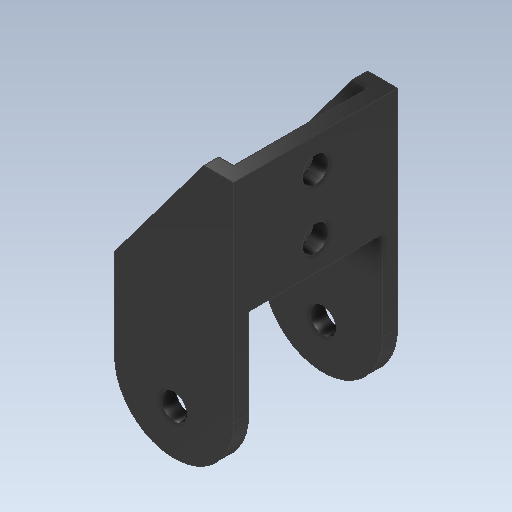
# Autodesk Inventor part: Kit de Sujeción 2
Saved by Autodesk Inventor 2020 (Build 240168000, 168)
## iProperties
Created: 2020-07-05
Part Number: Kit de Sujeción 2
Material: Genérico
Document SubType Name: Modeling
Designer: Pipi
Density: 1 g/cm^3
Appearance: Brillante - Negro
Author: Pipi
Autodesk Inventor part; units mm, degrees
ref_plane "YZ Plane" through (0, 0, 0) normal (1, 0, 0) x (0, 1, 0)
ref_plane "XZ Plane" through (0, 0, 0) normal (0, 1, 0) x (-1, 0, 0)
ref_plane "XY Plane" through (0, 0, 0) normal (0, 0, 1) x (1, 0, 0)
sketch "Boceto1" plane through (0, 0, 0) normal (0, 1, 0) x (-1, 0, 0)
  line L0 (10.3005, 0.2018) -> (-1.6995, 0.2018)
  line L1 (-1.6995, 0.2018) -> (-1.6995, 18.2018)
  line L2 (-1.6995, 18.2018) -> (10.3005, 18.2018)
  line L3 (12.3005, 20.2018) -> (-3.6995, 20.2018)
  line L4 (-3.6995, 20.2018) -> (-3.6995, -1.7982)
  line L5 (-3.6995, -1.7982) -> (12.3005, -1.7982)
  line L6 (10.3005, 18.2018) -> (12.3005, 18.2018)
  line L7 (10.3005, 0.2018) -> (12.3005, 0.2018)
  line L8 (12.3005, -1.7982) -> (12.3005, 0.2018)
  line L9 (12.3005, 18.2018) -> (12.3005, 20.2018)
  point P0 (0, 0)
  point P1 (0, 0)
  dimension "d0" = 18
  dimension "d1" = 12
  constraints: 20 end point, 10 perpendicular, 2 other
  measures "d0" distance of L2.end L0.start
  measures "d1" distance of L0.start L0.end
extrude "Extrusión1" add sketch "Boceto1" along normal blind 28
sketch "Boceto4" plane through (1.6995, 0, 0.2018) normal (-1, 0, 0) x (0, 0, 1)
  line L0 (18, 0) -> (18, 28) projected
  line L1 (18, 28) -> (18, 12)
  line L2 (18, 12) -> (0, 12)
  line L3 (0, 0) -> (0, 28) projected
  line L4 (18, 28) -> (0, 28)
  line L5 (0, 28) -> (0, 12)
  line L6 (20, 28) -> (-2, 28) projected
  line L7 (9, 28) -> (9, 12)
  circle A0 centre (9, 24) radius 1.75
  circle A1 centre (9, 16) radius 1.75
  line L8 (18, 12) -> (18, 0)
  line L9 (0, 0) -> (18, 0) projected
  line L10 (0, 0) -> (0, 12)
  line L11 (18, 0) -> (0, 0)
  point P0 (-0.2018, 0)
  dimension "d14" = 16
  dimension "d15" = 3.5
  dimension "d16" = 3.5
  dimension "d17" = 4
  dimension "d18" = 4
  constraints: 16 end point, 4 point on line, 3 perpendicular, 2 centre point, 2 collinear, 2 midpoint, 1 horizontal
  measures "d14" distance of L0.end L1.end
  measures "d15" diameter of A0
  measures "d16" diameter of A1
  measures "d17" distance from line of L2 A1.centre
  measures "d18" distance of L7.start A0.centre
extrude "Extrusión4" cut sketch "Boceto4" against normal blind 2 contours L9 L3 L2 L0 | A1 L7 | L7 A1 | A0 L7 | L7 A0
sketch "Boceto5" plane through (3.6995, 28, -1.7982) normal (0, 0, -1) x (-1, 0, 0)
  line L0 (0, -28) -> (0, 0) projected
  line L1 (0, 0) -> (4, 0)
  line L2 (16, 0) -> (0, 0) projected
  line L3 (0, 0) -> (0, -16)
  line L4 (0, -16) -> (16, -16)
  line L5 (16, -28) -> (16, 0) projected
  line L6 (4, 0) -> (16, -16)
  line L7 (4, 0) -> (4, -16)
  point P0 (3.6995, -28)
  point P1 (0, -26.5)
  point P2 (16, -26.5)
  dimension "d21" = 4
  dimension "d22" = 16
  constraints: 10 end point, 4 point on line, 2 perpendicular
  measures "d21" distance of L0.end L1.end
  measures "d22" distance of L0.end L3.end
extrude "Extrusión5" cut sketch "Boceto5" against normal blind 30 contours L2 L5 L6
sketch "Boceto6" plane through (3.6995, 0, -1.7982) normal (0, 0, -1) x (-1, 0, 0)
  line L0 (0, 12) -> (0, 0) projected
  line L1 (16, 0) -> (16, 12) projected
  arc A0 (0, 0) -> (16, 0) centre (8, -0.0553) ccw
  line L2 (16, 0) -> (0, 0) projected
  line L3 (16, 0) -> (0, 0)
  point P0 (3.6995, 0)
  constraints: 2 end point, 2 point on circle, 1 centre point, 1 horizontal
sketch "Boceto7" plane through (-12.3005, 0, 20.2018) normal (0, 0, 1) x (1, 0, 0)
  line L0 (0, 12) -> (0, 0)
  line L1 (16, 0) -> (16, 12)
  arc A0 (0, 0) -> (16, 0) centre (8, -0.0553) ccw
  line L2 (0, 0) -> (16, 0) projected
  line L3 (0, 0) -> (16, 0)
  circle A1 centre (8, -2.0553) radius 1.75
  point P0 (12.3005, 0)
  point P1 (3.6995, 0)
  dimension "d30" = 3.5
  dimension "d31" = 2
  constraints: 6 end point, 2 centre point, 2 point on circle, 1 collinear
  measures "d30" diameter of A1
  measures "d31" distance of A0.centre A1.centre
extrude "Extrusión6" add sketch "Boceto7" against normal blind 2 contours L2 A0 | A1
extrude "Extrusión7" add sketch "Boceto6" against normal blind 2
extrude "Extrusión8" cut sketch "Boceto7" against normal blind 30 contours A1
